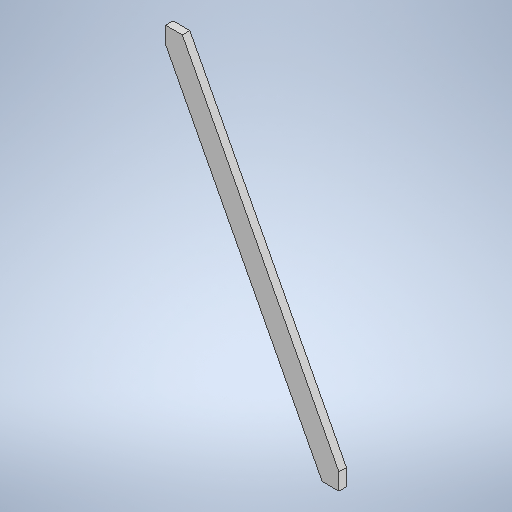
# Autodesk Inventor part: Support - Left
Saved by Autodesk Inventor 2025.2 (Build 292293000, 293)
## iProperties
Created: 2025-02-17
Part Number: Support - Left
Material: Generic
Document SubType Name: Modeling
Designer: baolo
Density: 1 g/cm^3
Appearance: Default
Author: baolo
Autodesk Inventor part; units mm, degrees
ref_plane "YZ Plane" through (0, 0, 0) normal (1, 0, 0) x (0, 1, 0)
ref_plane "XZ Plane" through (0, 0, 0) normal (0, 1, 0) x (-1, 0, 0)
ref_plane "XY Plane" through (0, 0, 0) normal (0, 0, 1) x (1, 0, 0)
sketch "Sketch1" plane through (0, 0, 0) normal (0, 0, 1) x (1, 0, 0)
  line L0 (-276.4159, 0) -> (46.0693, 0) construction
  line L1 (-22.2362, 22.2362) -> (0, 22.2362) construction
  line L2 (0, 22.2362) -> (0, 0)
  line L3 (0, 0) -> (-22.2362, 0)
  line L4 (-22.2362, 0) -> (-22.2362, 22.2362) construction
  line L5 (-22.2362, 22.2362) -> (0, 0) construction
  line L6 (0, 22.2362) -> (-22.2362, 0) construction
  line L7 (-230.3465, 421.1181) -> (-208.1103, 421.1181)
  line L8 (-208.1103, 421.1181) -> (-208.1103, 398.8819) construction
  line L9 (-208.1103, 398.8819) -> (-230.3465, 398.8819) construction
  line L10 (-230.3465, 398.8819) -> (-230.3465, 421.1181)
  line L11 (-230.3465, 421.1181) -> (-208.1103, 398.8819) construction
  line L12 (-208.1103, 421.1181) -> (-230.3465, 398.8819) construction
  line L13 (-230.3465, 398.8819) -> (-22.2362, 0)
  line L14 (-208.1103, 421.1181) -> (0, 22.2362)
  point P0 (-11.1181, 11.1181)
  point P1 (-219.2284, 410)
  dimension "d16" = 480
  dimension "d17" = 30
  dimension "d18" = 410
  constraints: 28 end point, 4 midpoint, 4 parallel, 3 equal length, 2 horizontal, 2 perpendicular
  measures "d16" distance of L2.end L7.start
  measures "d17" distance between parallel lines of L13 L14
  measures "d18" distance from line of L0 point (-219.228, 410)
extrude "Extrusion1" add sketch "Sketch1" along normal mid plane 10
body "Solid1"
